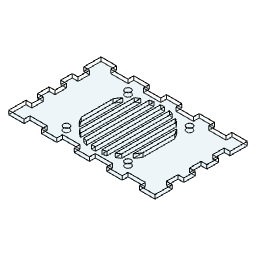
case_1_3mm (Autodesk Fusion 360 design; units mm, degrees)
Autodesk Fusion 360 part; units mm, degrees
sketch "スケッチ1" plane through (0, 0, 0) normal (0, 0, 1) x (1, 0, 0)
  line L0 (0, 0) -> (74, 0)
  line L1 (74, 0) -> (74, 46)
  line L2 (74, 46) -> (0, 46)
  line L3 (0, 46) -> (0, 0)
  dimension "d1" = 46
  dimension "d2" = 74
  constraint horizontal L0
  constraint vertical L1
  constraint horizontal L2
  constraint vertical L3
  constraint coincident L0.start L3.end
  measures "d1" distance of L0.start L2.end
  measures "d2" distance of L0.start L0.end
extrude "押し出し1" add sketch "スケッチ1" along normal blind 2
sketch "スケッチ2" plane through (0, 0, 2) normal (0, 0, 1) x (-1, 0, 0)
  line L0 (0, -46) -> (0, 0)
  line L1 (0, 0) -> (-74, 0)
  line L2 (-74, 0) -> (-74, -46)
  line L3 (-74, -46) -> (0, -46)
  circle A0 centre (-53, -39) radius 1.6
  circle A1 centre (-53, -39) radius 1.6
  circle A2 centre (-53, -7) radius 1.6
  circle A3 centre (-21, -7) radius 1.6
  circle A4 centre (-21, -39) radius 1.6
  dimension "d5" = 3.2
  dimension "d6" = 7
  dimension "d7" = 21
  dimension "d8" = 3.2
  dimension "d9" = 3.2
  dimension "d10" = 3.2
  dimension "d11" = 3.2
  dimension "d12" = 7
  dimension "d13" = 21
  measures "d5" diameter of A0
  measures "d6" distance of L3 A0.centre
  measures "d7" distance of L2 A0.centre
  measures "d8" diameter of A1
  measures "d9" diameter of A2
  measures "d10" diameter of A4
  measures "d11" diameter of A3
  measures "d12" distance of L3 A4.centre
  measures "d13" distance of L0 A4.centre
hole "穴1" at (21, 39, 2) at (53, 39, 2) at (53, 7, 2) at (21, 7, 2) direction (0, 0, -1) diameter 3.2 depth 16 tip angle 118
sketch "スケッチ3" plane through (0, 0, 2) normal (0, 0, 1) x (-1, 0, 0)
  circle A0 centre (-53, -7) radius 1.6
  circle A1 centre (-21, -39) radius 1.6
  circle A2 centre (-53, -39) radius 1.6
  circle A3 centre (-21, -7) radius 1.6
  line L0 (0, -46) -> (0, 0)
  line L1 (0, 0) -> (-74, 0)
  line L2 (-74, 0) -> (-74, -46)
  line L3 (-74, -46) -> (0, -46)
  line L4 (-58, -46) -> (-67, -46)
  line L5 (-67, -46) -> (-67, -44)
  line L6 (-67, -44) -> (-58, -44)
  line L7 (-58, -44) -> (-58, -46)
  line L8 (-50, -46) -> (-50, -44)
  line L9 (-41, -46) -> (-50, -46)
  line L10 (-50, -44) -> (-41, -44)
  line L11 (-41, -44) -> (-41, -46)
  line L12 (-33, -46) -> (-33, -44)
  line L13 (-24, -46) -> (-33, -46)
  line L14 (-33, -44) -> (-24, -44)
  line L15 (-24, -44) -> (-24, -46)
  line L16 (-16, -46) -> (-16, -44)
  line L17 (-7, -46) -> (-16, -46)
  line L18 (-16, -44) -> (-7, -44)
  line L19 (-7, -44) -> (-7, -46)
  line L20 (0, -38) -> (-2, -38)
  line L21 (-2, -38) -> (-2, -32)
  line L22 (-2, -32) -> (0, -32)
  line L23 (0, -32) -> (0, -38)
  line L24 (-2, -20) -> (0, -20)
  line L25 (0, -20) -> (0, -26)
  line L26 (-2, -26) -> (-2, -20)
  line L27 (0, -26) -> (-2, -26)
  line L28 (-2, -8) -> (0, -8)
  line L29 (0, -8) -> (0, -14)
  line L30 (-2, -14) -> (-2, -8)
  line L31 (0, -14) -> (-2, -14)
  line L32 (-72, -8) -> (-72, -14)
  line L33 (-72, -38) -> (-74, -38)
  line L34 (-72, -32) -> (-72, -38)
  line L35 (-74, -26) -> (-74, -20)
  line L36 (-74, -32) -> (-72, -32)
  line L37 (-74, -20) -> (-72, -20)
  line L38 (-72, -20) -> (-72, -26)
  line L39 (-74, -14) -> (-74, -8)
  line L40 (-72, -26) -> (-74, -26)
  line L41 (-74, -38) -> (-74, -32)
  line L42 (-74, -8) -> (-72, -8)
  line L43 (-72, -14) -> (-74, -14)
  line L44 (-144, -8) -> (-144, -14)
  line L45 (-144, -38) -> (-146, -38)
  line L46 (-144, -32) -> (-144, -38)
  line L47 (-146, -26) -> (-146, -20)
  line L48 (-146, -32) -> (-144, -32)
  line L49 (-146, -20) -> (-144, -20)
  line L50 (-144, -20) -> (-144, -26)
  line L51 (-146, -14) -> (-146, -8)
  line L52 (-144, -26) -> (-146, -26)
  line L53 (-146, -38) -> (-146, -32)
  line L54 (-146, -8) -> (-144, -8)
  line L55 (-144, -14) -> (-146, -14)
  line L56 (-41, 0) -> (-41, -2)
  line L57 (-67, 0) -> (-58, 0)
  line L58 (-67, -2) -> (-67, 0)
  line L59 (-41, -2) -> (-50, -2)
  line L60 (-7, 0) -> (-7, -2)
  line L61 (-24, 0) -> (-24, -2)
  line L62 (-33, 0) -> (-24, 0)
  line L63 (-50, -2) -> (-50, 0)
  line L64 (-24, -2) -> (-33, -2)
  line L65 (-7, -2) -> (-16, -2)
  line L66 (-58, -2) -> (-67, -2)
  line L67 (-16, -2) -> (-16, 0)
  line L68 (-50, 0) -> (-41, 0)
  line L69 (-58, 0) -> (-58, -2)
  line L70 (-16, 0) -> (-7, 0)
  line L71 (-33, -2) -> (-33, 0)
  line L72 (-41, 44) -> (-41, 42)
  line L73 (-67, 44) -> (-58, 44)
  line L74 (-67, 42) -> (-67, 44)
  line L75 (-41, 42) -> (-50, 42)
  line L76 (-7, 44) -> (-7, 42)
  line L77 (-24, 44) -> (-24, 42)
  line L78 (-33, 44) -> (-24, 44)
  line L79 (-50, 42) -> (-50, 44)
  line L80 (-24, 42) -> (-33, 42)
  line L81 (-7, 42) -> (-16, 42)
  line L82 (-58, 42) -> (-67, 42)
  line L83 (-16, 42) -> (-16, 44)
  line L84 (-50, 44) -> (-41, 44)
  line L85 (-58, 44) -> (-58, 42)
  line L86 (-16, 44) -> (-7, 44)
  line L87 (-33, 42) -> (-33, 44)
  dimension "d17" = 9
  dimension "d18" = 2
  dimension "d19" = 7
  dimension "d22" = 17
  dimension "d23" = 0
  dimension "d24" = 6
  dimension "d25" = 2
  dimension "d26" = 8
  dimension "d29" = 0
  dimension "d30" = 12
  dimension "d33" = -72
  dimension "d34" = 0
  dimension "d37" = 0
  dimension "d38" = 44
  constraint horizontal L4
  constraint vertical L5
  constraint horizontal L6
  constraint vertical L7
  constraint coincident L3 L4.start
  constraint horizontal L20
  constraint vertical L21
  constraint horizontal L22
  constraint vertical L23
  constraint coincident L0 L20.start
  measures "d17" distance of L5.end L6.end
  measures "d18" distance of L4.end L5.end
  measures "d19" distance of L2 L5
  measures "d24" distance of L20.start L22.end
  measures "d25" distance of L20.start L20.end
  measures "d26" distance of L3 L20.start
extrude "押し出し2" cut sketch "スケッチ3" against normal blind 2 contours L0 L20 L21 L22 L23 | L3 L16 L17 L18 L19 | L0 L24 L25 L26 L27 | L3 L12 L13 L14 L15 | L0 L28 L29 L30 L31 | L3 L8 L9 L10 L11 | L3 L4 L5 L6 L7 | L1 L60 L65 L67 L70 | L1 L61 L62 L64 L71 | L2 L33 L34 L36 L41 | L1 L56 L59 L63 L68 | L2 L35 L37 L38 L40 | L1 L57 L58 L66 L69 | L2 L32 L39 L42 L43
sketch "スケッチ4" plane through (0, 0, 2) normal (0, 0, 1) x (-1, 0, 0)
  line L0 (-50, -2) -> (-50, 0)
  line L1 (-50, 0) -> (-58, 0)
  line L2 (-58, 0) -> (-58, -2)
  line L3 (-58, -2) -> (-67, -2)
  line L4 (-67, -2) -> (-67, 0)
  line L5 (-67, 0) -> (-74, 0)
  line L6 (-74, 0) -> (-74, -8)
  line L7 (-74, -8) -> (-72, -8)
  line L8 (-72, -8) -> (-72, -14)
  line L9 (-72, -14) -> (-74, -14)
  line L10 (-74, -14) -> (-74, -20)
  line L11 (-74, -20) -> (-72, -20)
  line L12 (-72, -20) -> (-72, -26)
  line L13 (-72, -26) -> (-74, -26)
  line L14 (-74, -26) -> (-74, -32)
  line L15 (-74, -32) -> (-72, -32)
  line L16 (-72, -32) -> (-72, -38)
  line L17 (-72, -38) -> (-74, -38)
  line L18 (-74, -38) -> (-74, -46)
  line L19 (-74, -46) -> (-67, -46)
  line L20 (-67, -46) -> (-67, -44)
  line L21 (-67, -44) -> (-58, -44)
  line L22 (-58, -44) -> (-58, -46)
  line L23 (-58, -46) -> (-50, -46)
  line L24 (-50, -46) -> (-50, -44)
  line L25 (-50, -44) -> (-41, -44)
  line L26 (-41, -44) -> (-41, -46)
  line L27 (-41, -46) -> (-33, -46)
  line L28 (-33, -46) -> (-33, -44)
  line L29 (-33, -44) -> (-24, -44)
  line L30 (-24, -44) -> (-24, -46)
  line L31 (-24, -46) -> (-16, -46)
  line L32 (-16, -46) -> (-16, -44)
  line L33 (-16, -44) -> (-7, -44)
  line L34 (-7, -44) -> (-7, -46)
  line L35 (-7, -46) -> (0, -46)
  line L36 (0, -46) -> (0, -38)
  line L37 (0, -38) -> (-2, -38)
  line L38 (-2, -38) -> (-2, -32)
  line L39 (-2, -32) -> (0, -32)
  line L40 (0, -32) -> (0, -26)
  line L41 (0, -26) -> (-2, -26)
  line L42 (-2, -26) -> (-2, -20)
  line L43 (-2, -20) -> (0, -20)
  line L44 (0, -20) -> (0, -14)
  line L45 (0, -14) -> (-2, -14)
  line L46 (-2, -14) -> (-2, -8)
  line L47 (-2, -8) -> (0, -8)
  line L48 (0, -8) -> (0, 0)
  line L49 (0, 0) -> (-7, 0)
  line L50 (-7, 0) -> (-7, -2)
  line L51 (-7, -2) -> (-16, -2)
  line L52 (-16, -2) -> (-16, 0)
  line L53 (-16, 0) -> (-24, 0)
  line L54 (-24, 0) -> (-24, -2)
  line L55 (-24, -2) -> (-33, -2)
  line L56 (-33, -2) -> (-33, 0)
  line L57 (-33, 0) -> (-41, 0)
  line L58 (-41, 0) -> (-41, -2)
  line L59 (-41, -2) -> (-50, -2)
  circle A0 centre (-53, -7) radius 1.6
  circle A1 centre (-21, -39) radius 1.6
  circle A2 centre (-53, -39) radius 1.6
  circle A3 centre (-21, -7) radius 1.6
  circle A4 centre (-37, -23) radius 18
  line L60 (-36, -42) -> (-38, -42)
  line L61 (-38, -42) -> (-38, -4)
  line L62 (-38, -4) -> (-36, -4)
  line L63 (-36, -4) -> (-36, -42)
  line L64 (-41, -42) -> (-43, -42)
  line L65 (-43, -42) -> (-43, -5)
  line L66 (-43, -5) -> (-41, -5)
  line L67 (-41, -5) -> (-41, -42)
  line L68 (-46, -40) -> (-48, -40)
  line L69 (-48, -40) -> (-48, -6)
  line L70 (-48, -6) -> (-46, -6)
  line L71 (-46, -6) -> (-46, -40)
  line L72 (-51, -36) -> (-53, -36)
  line L73 (-53, -36) -> (-53, -11)
  line L74 (-53, -11) -> (-51, -11)
  line L75 (-51, -11) -> (-51, -36)
  line L76 (-33, -42) -> (-31, -42)
  line L77 (-31, -42) -> (-31, -4)
  line L78 (-31, -4) -> (-33, -4)
  line L79 (-33, -4) -> (-33, -42)
  line L80 (-28, -40) -> (-26, -40)
  line L81 (-26, -40) -> (-26, -6)
  line L82 (-26, -6) -> (-28, -6)
  line L83 (-28, -6) -> (-28, -40)
  line L84 (-23, -36) -> (-21, -36)
  line L85 (-21, -36) -> (-21, -11)
  line L86 (-21, -11) -> (-23, -11)
  line L87 (-23, -11) -> (-23, -36)
  constraint horizontal L60
  constraint vertical L61
  constraint horizontal L62
  constraint vertical L63
  constraint horizontal L64
  constraint vertical L65
  constraint horizontal L66
  constraint vertical L67
  constraint horizontal L68
  constraint vertical L69
  constraint horizontal L70
  constraint vertical L71
  constraint horizontal L72
  constraint vertical L73
  constraint horizontal L74
  constraint vertical L75
  constraint horizontal L76
  constraint vertical L77
  constraint horizontal L78
  constraint vertical L79
  constraint horizontal L80
  constraint vertical L81
  constraint horizontal L82
  constraint vertical L83
  constraint horizontal L84
  constraint vertical L85
  constraint horizontal L86
  constraint vertical L87
extrude "押し出し3" cut sketch "スケッチ4" against normal blind 2 contours A4 L85 L87 | A4 L81 L83 | A4 L77 L79 | A4 L61 L63 | A4 L65 L67 | A4 L69 L71 | A4 L73 L75
sketch "スケッチ5" plane through (0, 0, 2) normal (0, 0, 1) x (-1, 0, 0)
  line L0 (-33, -40.5499) -> (-33, -5.4501)
  arc A0 (-31, -6.0294) -> (-33, -5.4501) centre (-37, -23) ccw
  line L1 (-31, -6.0294) -> (-31, -39.9706)
  arc A1 (-33, -40.5499) -> (-31, -39.9706) centre (-37, -23) ccw
  line L2 (-51, -11.6863) -> (-51, -34.3137)
  arc A2 (-53, -31.2462) -> (-51, -34.3137) centre (-37, -23) ccw
  line L3 (-53, -31.2462) -> (-53, -14.7538)
  arc A3 (-51, -11.6863) -> (-53, -14.7538) centre (-37, -23) ccw
  line L4 (-36, -5.0278) -> (-36, -40.9722)
  arc A4 (-38, -40.9722) -> (-36, -40.9722) centre (-37, -23) ccw
  line L5 (-38, -40.9722) -> (-38, -5.0278)
  arc A5 (-36, -5.0278) -> (-38, -5.0278) centre (-37, -23) ccw
  line L6 (-28, -38.5885) -> (-28, -7.4115)
  arc A6 (-26, -8.7522) -> (-28, -7.4115) centre (-37, -23) ccw
  line L7 (-26, -8.7522) -> (-26, -37.2478)
  arc A7 (-28, -38.5885) -> (-26, -37.2478) centre (-37, -23) ccw
  line L8 (-46, -7.4115) -> (-46, -38.5885)
  arc A8 (-48, -37.2478) -> (-46, -38.5885) centre (-37, -23) ccw
  line L9 (-48, -37.2478) -> (-48, -8.7522)
  arc A9 (-46, -7.4115) -> (-48, -8.7522) centre (-37, -23) ccw
  line L10 (-41, -5.4501) -> (-41, -40.5499)
  arc A10 (-43, -39.9706) -> (-41, -40.5499) centre (-37, -23) ccw
  line L11 (-43, -39.9706) -> (-43, -6.0294)
  arc A11 (-41, -5.4501) -> (-43, -6.0294) centre (-37, -23) ccw
  line L12 (-23, -34.3137) -> (-23, -11.6863)
  arc A12 (-21, -14.7538) -> (-23, -11.6863) centre (-37, -23) ccw
  line L13 (-21, -14.7538) -> (-21, -31.2462)
  arc A13 (-23, -34.3137) -> (-21, -31.2462) centre (-37, -23) ccw
  line L14 (-50, -2) -> (-50, 0)
  line L15 (-50, 0) -> (-58, 0)
  line L16 (-58, 0) -> (-58, -2)
  line L17 (-58, -2) -> (-67, -2)
  line L18 (-67, -2) -> (-67, 0)
  line L19 (-67, 0) -> (-74, 0)
  line L20 (-74, 0) -> (-74, -8)
  line L21 (-74, -8) -> (-72, -8)
  line L22 (-72, -8) -> (-72, -14)
  line L23 (-72, -14) -> (-74, -14)
  line L24 (-74, -14) -> (-74, -20)
  line L25 (-74, -20) -> (-72, -20)
  line L26 (-72, -20) -> (-72, -26)
  line L27 (-72, -26) -> (-74, -26)
  line L28 (-74, -26) -> (-74, -32)
  line L29 (-74, -32) -> (-72, -32)
  line L30 (-72, -32) -> (-72, -38)
  line L31 (-72, -38) -> (-74, -38)
  line L32 (-74, -38) -> (-74, -46)
  line L33 (-74, -46) -> (-67, -46)
  line L34 (-67, -46) -> (-67, -44)
  line L35 (-67, -44) -> (-58, -44)
  line L36 (-58, -44) -> (-58, -46)
  line L37 (-58, -46) -> (-50, -46)
  line L38 (-50, -46) -> (-50, -44)
  line L39 (-50, -44) -> (-41, -44)
  line L40 (-41, -44) -> (-41, -46)
  line L41 (-41, -46) -> (-33, -46)
  line L42 (-33, -46) -> (-33, -44)
  line L43 (-33, -44) -> (-24, -44)
  line L44 (-24, -44) -> (-24, -46)
  line L45 (-24, -46) -> (-16, -46)
  line L46 (-16, -46) -> (-16, -44)
  line L47 (-16, -44) -> (-7, -44)
  line L48 (-7, -44) -> (-7, -46)
  line L49 (-7, -46) -> (0, -46)
  line L50 (0, -46) -> (0, -38)
  line L51 (0, -38) -> (-2, -38)
  line L52 (-2, -38) -> (-2, -32)
  line L53 (-2, -32) -> (0, -32)
  line L54 (0, -32) -> (0, -26)
  line L55 (0, -26) -> (-2, -26)
  line L56 (-2, -26) -> (-2, -20)
  line L57 (-2, -20) -> (0, -20)
  line L58 (0, -20) -> (0, -14)
  line L59 (0, -14) -> (-2, -14)
  line L60 (-2, -14) -> (-2, -8)
  line L61 (-2, -8) -> (0, -8)
  line L62 (0, -8) -> (0, 0)
  line L63 (0, 0) -> (-7, 0)
  line L64 (-7, 0) -> (-7, -2)
  line L65 (-7, -2) -> (-16, -2)
  line L66 (-16, -2) -> (-16, 0)
  line L67 (-16, 0) -> (-24, 0)
  line L68 (-24, 0) -> (-24, -2)
  line L69 (-24, -2) -> (-33, -2)
  line L70 (-33, -2) -> (-33, 0)
  line L71 (-33, 0) -> (-41, 0)
  line L72 (-41, 0) -> (-41, -2)
  line L73 (-41, -2) -> (-50, -2)
  circle A14 centre (-53, -7) radius 1.6
  circle A15 centre (-21, -39) radius 1.6
  circle A16 centre (-53, -39) radius 1.6
  circle A17 centre (-21, -7) radius 1.6
  line L74 (0, 0) -> (-7, 0)
  line L75 (-7, 0) -> (-7, 1)
  line L76 (-7, 1) -> (0, 1)
  line L77 (0, 1) -> (0, 0)
  line L78 (-16, 0) -> (-24, 0)
  line L79 (-24, 0) -> (-24, 1)
  line L80 (-24, 1) -> (-16, 1)
  line L81 (-16, 1) -> (-16, 0)
  line L82 (-33, 0) -> (-41, 0)
  line L83 (-41, 0) -> (-41, 1)
  line L84 (-41, 1) -> (-33, 1)
  line L85 (-33, 1) -> (-33, 0)
  line L86 (-50, 0) -> (-58, 0)
  line L87 (-58, 0) -> (-58, 1)
  line L88 (-58, 1) -> (-50, 1)
  line L89 (-50, 1) -> (-50, 0)
  line L90 (-67, 0) -> (-75, 0)
  line L91 (-75, 0) -> (-75, 1)
  line L92 (-75, 1) -> (-67, 1)
  line L93 (-67, 1) -> (-67, 0)
  line L94 (-74, 0) -> (-75, 0)
  line L95 (-75, 0) -> (-75, -8)
  line L96 (-75, -8) -> (-74, -8)
  line L97 (-74, -8) -> (-74, 0)
  line L98 (-74, -14) -> (-75, -14)
  line L99 (-75, -14) -> (-75, -20)
  line L100 (-75, -20) -> (-74, -20)
  line L101 (-74, -20) -> (-74, -14)
  line L102 (-74, -26) -> (-75, -26)
  line L103 (-75, -26) -> (-75, -32)
  line L104 (-75, -32) -> (-74, -32)
  line L105 (-74, -32) -> (-74, -26)
  line L106 (-74, -38) -> (-75, -38)
  line L107 (-75, -38) -> (-75, -46)
  line L108 (-75, -46) -> (-74, -46)
  line L109 (-74, -46) -> (-74, -38)
  line L110 (-67, -46) -> (-75, -46)
  line L111 (-75, -46) -> (-75, -47)
  line L112 (-75, -47) -> (-67, -47)
  line L113 (-67, -47) -> (-67, -46)
  line L114 (-58, -46) -> (-50, -46)
  line L115 (-50, -46) -> (-50, -47)
  line L116 (-50, -47) -> (-58, -47)
  line L117 (-58, -47) -> (-58, -46)
  line L118 (-41, -46) -> (-33, -46)
  line L119 (-33, -46) -> (-33, -47)
  line L120 (-33, -47) -> (-41, -47)
  line L121 (-41, -47) -> (-41, -46)
  line L122 (-24, -46) -> (-16, -46)
  line L123 (-16, -46) -> (-16, -47)
  line L124 (-16, -47) -> (-24, -47)
  line L125 (-24, -47) -> (-24, -46)
  line L126 (-7, -46) -> (0, -46)
  line L127 (0, -46) -> (0, -47)
  line L128 (0, -47) -> (-7, -47)
  line L129 (-7, -47) -> (-7, -46)
  line L130 (1, -47) -> (0, -47)
  line L131 (0, -47) -> (0, -38)
  line L132 (0, -38) -> (1, -38)
  line L133 (1, -38) -> (1, -47)
  line L134 (1, -32) -> (0, -32)
  line L135 (0, -32) -> (0, -26)
  line L136 (0, -26) -> (1, -26)
  line L137 (1, -26) -> (1, -32)
  line L138 (1, -20) -> (0, -20)
  line L139 (0, -20) -> (0, -14)
  line L140 (0, -14) -> (1, -14)
  line L141 (1, -14) -> (1, -20)
  line L142 (1, -8) -> (0, -8)
  line L143 (0, -8) -> (0, 1)
  line L144 (0, 1) -> (1, 1)
  line L145 (1, 1) -> (1, -8)
  constraint horizontal L74
  constraint vertical L75
  constraint horizontal L76
  constraint vertical L77
  constraint coincident L62.end L63.start
  constraint horizontal L78
  constraint vertical L79
  constraint horizontal L80
  constraint vertical L81
  constraint coincident L66.end L67.start
  constraint horizontal L82
  constraint vertical L83
  constraint horizontal L84
  constraint vertical L85
  constraint coincident L70.end L71.start
  constraint horizontal L86
  constraint vertical L87
  constraint horizontal L88
  constraint vertical L89
  constraint coincident L14.end L15.start
  constraint horizontal L90
  constraint vertical L91
  constraint horizontal L92
  constraint vertical L93
  constraint coincident L18.end L19.start
  constraint horizontal L94
  constraint vertical L95
  constraint horizontal L96
  constraint vertical L97
  constraint coincident L19.end L20.start
  constraint horizontal L98
  constraint vertical L99
  constraint horizontal L100
  constraint vertical L101
  constraint coincident L23.end L24.start
  constraint horizontal L102
  constraint vertical L103
  constraint horizontal L104
  constraint vertical L105
  constraint coincident L27.end L28.start
  constraint horizontal L106
  constraint vertical L107
  constraint horizontal L108
  constraint vertical L109
  constraint coincident L31.end L32.start
  constraint horizontal L110
  constraint vertical L111
  constraint horizontal L112
  constraint vertical L113
  constraint coincident L33.end L34.start
  constraint horizontal L114
  constraint vertical L115
  constraint horizontal L116
  constraint vertical L117
  constraint coincident L36.end L37.start
  constraint horizontal L118
  constraint vertical L119
  constraint horizontal L120
  constraint vertical L121
  constraint coincident L40.end L41.start
  constraint horizontal L122
  constraint vertical L123
  constraint horizontal L124
  constraint vertical L125
  constraint coincident L44.end L45.start
  constraint horizontal L126
  constraint vertical L127
  constraint horizontal L128
  constraint vertical L129
  constraint coincident L48.end L49.start
  constraint horizontal L130
  constraint vertical L131
  constraint horizontal L132
  constraint vertical L133
  constraint coincident L50.end L51.start
  constraint horizontal L134
  constraint vertical L135
  constraint horizontal L136
  constraint vertical L137
  constraint coincident L54.end L55.start
  constraint horizontal L138
  constraint vertical L139
  constraint horizontal L140
  constraint vertical L141
  constraint coincident L58.end L59.start
  constraint horizontal L142
  constraint vertical L143
  constraint horizontal L144
  constraint vertical L145
extrude "押し出し4" add sketch "スケッチ5" against normal blind 2 contours L15 L86 L87 L88 L89 | L71 L82 L83 L84 L85 | L19 L90 L91 L92 L93 L94 | L20 L90 L94 L95 L96 L97 | L67 L78 L79 L80 L81 | L24 L98 L99 L100 L101 | L63 L74 L75 L76 L77 L143 | L62 L77 L142 L143 L144 L145 | L28 L102 L103 L104 L105 | L58 L138 L139 L140 L141 | L32 L106 L107 L108 L109 L110 | L33 L108 L110 L111 L112 L113 | L54 L134 L135 L136 L137 | L37 L114 L115 L116 L117 | L50 L127 L130 L131 L132 L133 | L49 L126 L127 L128 L129 L131 | L41 L118 L119 L120 L121 | L45 L122 L123 L124 L125
sketch "スケッチ6" plane through (0, 0, 0) normal (0, 0, -1) x (1, 0, 0)
  line L0 (33, -5.4501) -> (33, -40.5499)
  arc A0 (31, -39.9706) -> (33, -40.5499) centre (37, -23) ccw
  line L1 (31, -39.9706) -> (31, -6.0294)
  arc A1 (33, -5.4501) -> (31, -6.0294) centre (37, -23) ccw
  line L2 (51, -34.3137) -> (51, -11.6863)
  arc A2 (53, -14.7538) -> (51, -11.6863) centre (37, -23) ccw
  line L3 (53, -14.7538) -> (53, -31.2462)
  arc A3 (51, -34.3137) -> (53, -31.2462) centre (37, -23) ccw
  line L4 (36, -40.9722) -> (36, -5.0278)
  arc A4 (38, -5.0278) -> (36, -5.0278) centre (37, -23) ccw
  line L5 (38, -5.0278) -> (38, -40.9722)
  arc A5 (36, -40.9722) -> (38, -40.9722) centre (37, -23) ccw
  line L6 (28, -7.4115) -> (28, -38.5885)
  arc A6 (26, -37.2478) -> (28, -38.5885) centre (37, -23) ccw
  line L7 (26, -37.2478) -> (26, -8.7522)
  arc A7 (28, -7.4115) -> (26, -8.7522) centre (37, -23) ccw
  line L8 (46, -38.5885) -> (46, -7.4115)
  arc A8 (48, -8.7522) -> (46, -7.4115) centre (37, -23) ccw
  line L9 (48, -8.7522) -> (48, -37.2478)
  arc A9 (46, -38.5885) -> (48, -37.2478) centre (37, -23) ccw
  line L10 (41, -40.5499) -> (41, -5.4501)
  arc A10 (43, -6.0294) -> (41, -5.4501) centre (37, -23) ccw
  line L11 (43, -6.0294) -> (43, -39.9706)
  arc A11 (41, -40.5499) -> (43, -39.9706) centre (37, -23) ccw
  line L12 (23, -11.6863) -> (23, -34.3137)
  arc A12 (21, -31.2462) -> (23, -34.3137) centre (37, -23) ccw
  line L13 (21, -31.2462) -> (21, -14.7538)
  arc A13 (23, -11.6863) -> (21, -14.7538) centre (37, -23) ccw
  line L14 (50, 1) -> (50, -2)
  line L15 (50, -2) -> (41, -2)
  line L16 (41, -2) -> (41, 1)
  line L17 (41, 1) -> (33, 1)
  line L18 (33, 1) -> (33, -2)
  line L19 (33, -2) -> (24, -2)
  line L20 (24, -2) -> (24, 1)
  line L21 (24, 1) -> (16, 1)
  line L22 (16, 1) -> (16, -2)
  line L23 (16, -2) -> (7, -2)
  line L24 (7, -2) -> (7, 1)
  line L25 (7, 1) -> (-1, 1)
  line L26 (-1, 1) -> (-1, -8)
  line L27 (-1, -8) -> (2, -8)
  line L28 (2, -8) -> (2, -14)
  line L29 (2, -14) -> (-1, -14)
  line L30 (-1, -14) -> (-1, -20)
  line L31 (-1, -20) -> (2, -20)
  line L32 (2, -20) -> (2, -26)
  line L33 (2, -26) -> (-1, -26)
  line L34 (-1, -26) -> (-1, -32)
  line L35 (-1, -32) -> (2, -32)
  line L36 (2, -32) -> (2, -38)
  line L37 (2, -38) -> (-1, -38)
  line L38 (-1, -38) -> (-1, -47)
  line L39 (-1, -47) -> (7, -47)
  line L40 (7, -47) -> (7, -44)
  line L41 (7, -44) -> (16, -44)
  line L42 (16, -44) -> (16, -47)
  line L43 (16, -47) -> (24, -47)
  line L44 (24, -47) -> (24, -44)
  line L45 (24, -44) -> (33, -44)
  line L46 (33, -44) -> (33, -47)
  line L47 (33, -47) -> (41, -47)
  line L48 (41, -47) -> (41, -44)
  line L49 (41, -44) -> (50, -44)
  line L50 (50, -44) -> (50, -47)
  line L51 (50, -47) -> (58, -47)
  line L52 (58, -47) -> (58, -44)
  line L53 (58, -44) -> (67, -44)
  line L54 (67, -44) -> (67, -47)
  line L55 (67, -47) -> (75, -47)
  line L56 (75, -47) -> (75, -38)
  line L57 (75, -38) -> (72, -38)
  line L58 (72, -38) -> (72, -32)
  line L59 (72, -32) -> (75, -32)
  line L60 (75, -32) -> (75, -26)
  line L61 (75, -26) -> (72, -26)
  line L62 (72, -26) -> (72, -20)
  line L63 (72, -20) -> (75, -20)
  line L64 (75, -20) -> (75, -14)
  line L65 (75, -14) -> (72, -14)
  line L66 (72, -14) -> (72, -8)
  line L67 (72, -8) -> (75, -8)
  line L68 (75, -8) -> (75, 1)
  line L69 (75, 1) -> (67, 1)
  line L70 (67, 1) -> (67, -2)
  line L71 (67, -2) -> (58, -2)
  line L72 (58, -2) -> (58, 1)
  line L73 (58, 1) -> (50, 1)
  circle A14 centre (21, -7) radius 1.6
  circle A15 centre (53, -39) radius 1.6
  circle A16 centre (21, -39) radius 1.6
  circle A17 centre (53, -7) radius 1.6
